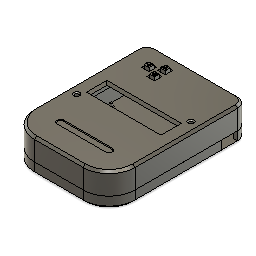
EqMountControllerCase (Autodesk Fusion 360 design; units mm, degrees)
Autodesk Fusion 360 part; units mm, degrees
sketch "Sketch1" plane through (0, 0, 0) normal (0, 1, 0) x (1, 0, 0)
  line L0 (0, 0) -> (75, 0) construction
  circle A0 centre (75, 0) radius 1.25
  line L1 (3, 0) -> (3, 29) construction
  line L2 (3, 29) -> (59, 29) construction
  line L3 (59, 29) -> (59, 65) construction
  line L4 (59, 65) -> (3, 65) construction
  line L5 (3, 65) -> (3, 29) construction
  circle A1 centre (3, 29) radius 1
  circle A2 centre (59, 29) radius 1
  circle A3 centre (59, 65) radius 1
  circle A4 centre (3, 65) radius 1
  line L6 (0, 0) -> (0, 31) construction
  line L7 (75, 0) -> (75, 31) construction
  line L8 (59, 65) -> (3, 29) construction
  line L9 (3, 65) -> (59, 29) construction
  line L10 (75, 31) -> (0, 0) construction
  line L11 (0, 31) -> (75, 0) construction
  line L12 (77.5, 33.5) -> (-2.5, 33.5) construction
  line L13 (-2.5, 33.5) -> (-2.5, -2.5) construction
  line L14 (-2.5, -2.5) -> (77.5, -2.5) construction
  line L15 (77.5, -2.5) -> (77.5, 33.5) construction
  line L16 (77.5, 33.5) -> (-2.5, -2.5) construction
  line L17 (-2.5, 33.5) -> (77.5, -2.5) construction
  line L18 (61, 67) -> (1, 67) construction
  line L19 (1, 67) -> (1, 27) construction
  line L20 (1, 27) -> (61, 27) construction
  line L21 (61, 27) -> (61, 67) construction
  line L22 (61, 67) -> (1, 27) construction
  line L23 (1, 67) -> (61, 27) construction
  line L24 (70, 8) -> (5, 8)
  line L25 (5, 8) -> (5, 23)
  line L26 (5, 23) -> (70, 23)
  line L27 (70, 23) -> (70, 8)
  line L28 (70, 8) -> (5, 23) construction
  line L29 (5, 8) -> (70, 23) construction
  line L30 (0, 70) -> (75, 70)
  line L31 (80, 65) -> (80, -30)
  line L32 (60, -50) -> (15, -50)
  line L33 (-5, -30) -> (-5, 65)
  arc A5 (80, 65) -> (75, 70) centre (75, 65) ccw
  arc A6 (0, 70) -> (-5, 65) centre (0, 65) ccw
  arc A7 (-5, -30) -> (15, -50) centre (15, -30) ccw
  arc A8 (60, -50) -> (80, -30) centre (60, -30) ccw
  arc A9 (0, 72) -> (-7, 65) centre (0, 65) ccw
  line L34 (-7, -30) -> (-7, 65)
  arc A10 (-7, -30) -> (15, -52) centre (15, -30) ccw
  line L35 (60, -52) -> (15, -52)
  arc A11 (60, -52) -> (82, -30) centre (60, -30) ccw
  line L36 (82, 65) -> (82, -30)
  arc A12 (82, 65) -> (75, 72) centre (75, 65) ccw
  line L37 (0, 72) -> (75, 72)
  arc A13 (0, 74) -> (-9, 65) centre (0, 65) ccw
  line L38 (-9, -30) -> (-9, 65)
  arc A14 (-9, -30) -> (15, -54) centre (15, -30) ccw
  line L39 (60, -54) -> (15, -54)
  arc A15 (60, -54) -> (84, -30) centre (60, -30) ccw
  line L40 (84, 65) -> (84, -30)
  arc A16 (84, 65) -> (75, 74) centre (75, 65) ccw
  line L41 (0, 74) -> (75, 74)
  line L42 (1, 67) -> (22, 67) construction
  line L43 (22, 67) -> (22, 60) construction
  line L44 (24.5, 57.5) -> (19.5, 57.5)
  line L45 (19.5, 57.5) -> (19.5, 62.5)
  line L46 (19.5, 62.5) -> (24.5, 62.5)
  line L47 (24.5, 62.5) -> (24.5, 57.5)
  line L48 (24.5, 57.5) -> (19.5, 62.5) construction
  line L49 (19.5, 57.5) -> (24.5, 62.5) construction
  line L50 (22, 67) -> (22, 50) construction
  line L51 (24.5, 47.5) -> (19.5, 47.5)
  line L52 (19.5, 47.5) -> (19.5, 52.5)
  line L53 (19.5, 52.5) -> (24.5, 52.5)
  line L54 (24.5, 52.5) -> (24.5, 47.5)
  line L55 (24.5, 47.5) -> (19.5, 52.5) construction
  line L56 (19.5, 47.5) -> (24.5, 52.5) construction
  line L57 (1, 67) -> (12, 67) construction
  line L58 (9.5, 52.5) -> (14.5, 52.5)
  line L59 (14.5, 52.5) -> (14.5, 57.5)
  line L60 (14.5, 57.5) -> (9.5, 57.5)
  line L61 (9.5, 57.5) -> (9.5, 52.5)
  line L62 (9.5, 52.5) -> (14.5, 57.5) construction
  line L63 (14.5, 52.5) -> (9.5, 57.5) construction
  circle A17 centre (3, 65) radius 2
  circle A18 centre (59, 65) radius 2
  circle A19 centre (59, 29) radius 2
  circle A20 centre (3, 29) radius 2
  circle A21 centre (75, 31) radius 3
  circle A22 centre (75, 0) radius 3
  circle A23 centre (0, 0) radius 3
  line L64 (84, 65) -> (80, 65)
  line L65 (80, 65) -> (80, 50)
  line L66 (80, 50) -> (84, 50)
  line L67 (84, 50) -> (84, 65)
  line L68 (-9, 65) -> (-5, 65)
  line L69 (-5, 65) -> (-5, 50)
  line L70 (-5, 50) -> (-9, 50)
  line L71 (-9, 50) -> (-9, 65)
  line L72 (26, 46) -> (8, 46)
  line L73 (8, 46) -> (8, 64)
  line L74 (8, 64) -> (26, 64)
  line L75 (26, 64) -> (26, 46)
  circle A24 centre (75, 31) radius 1.75
  circle A25 centre (0, 0) radius 1.75
  line L76 (8.5, 51.5) -> (15.5, 51.5)
  line L77 (15.5, 51.5) -> (15.5, 58.5)
  line L78 (15.5, 58.5) -> (8.5, 58.5)
  line L79 (8.5, 58.5) -> (8.5, 51.5)
  line L80 (25.5, 63.5) -> (25.5, 56.5)
  line L81 (25.5, 56.5) -> (18.5, 56.5)
  line L82 (18.5, 56.5) -> (18.5, 63.5)
  line L83 (18.5, 63.5) -> (25.5, 63.5)
  line L84 (25.5, 46.5) -> (18.5, 46.5)
  line L85 (18.5, 46.5) -> (18.5, 53.5)
  line L86 (18.5, 53.5) -> (25.5, 53.5)
  line L87 (25.5, 53.5) -> (25.5, 46.5)
  line L88 (9.7, 52.7) -> (14.3, 52.7)
  line L89 (14.3, 52.7) -> (14.3, 57.3)
  line L90 (14.3, 57.3) -> (9.7, 57.3)
  line L91 (9.7, 57.3) -> (9.7, 52.7)
  line L92 (24.3, 57.7) -> (19.7, 57.7)
  line L93 (19.7, 57.7) -> (19.7, 62.3)
  line L94 (19.7, 62.3) -> (24.3, 62.3)
  line L95 (24.3, 62.3) -> (24.3, 57.7)
  line L96 (24.3, 47.7) -> (19.7, 47.7)
  line L97 (19.7, 47.7) -> (19.7, 52.3)
  line L98 (19.7, 52.3) -> (24.3, 52.3)
  line L99 (24.3, 52.3) -> (24.3, 47.7)
  line L100 (9.7, 55) -> (13.15, 53.0081)
  line L101 (13.15, 53.0081) -> (13.15, 56.9919)
  line L102 (13.15, 56.9919) -> (9.7, 55)
  line L103 (22, 62.3) -> (20.0081, 58.85)
  line L104 (20.0081, 58.85) -> (23.9919, 58.85)
  line L105 (23.9919, 58.85) -> (22, 62.3)
  line L106 (22, 47.7) -> (23.9919, 51.15)
  line L107 (23.9919, 51.15) -> (20.0081, 51.15)
  line L108 (20.0081, 51.15) -> (22, 47.7)
  line L109 (76.25, 32.25) -> (73.75, 32.25)
  line L110 (73.75, 32.25) -> (73.75, 29.75)
  line L111 (73.75, 29.75) -> (76.25, 29.75)
  line L112 (76.25, 29.75) -> (76.25, 32.25)
  line L113 (76.25, 32.25) -> (73.75, 29.75) construction
  line L114 (73.75, 32.25) -> (76.25, 29.75) construction
  line L115 (1.25, 1.25) -> (-1.25, 1.25)
  line L116 (-1.25, 1.25) -> (-1.25, -1.25)
  line L117 (-1.25, -1.25) -> (1.25, -1.25)
  line L118 (1.25, -1.25) -> (1.25, 1.25)
  line L119 (1.25, 1.25) -> (-1.25, -1.25) construction
  line L120 (-1.25, 1.25) -> (1.25, -1.25) construction
  dimension "d2" = 75
  dimension "d3" = 2.5
  dimension "d4" = 29
  dimension "d5" = 56
  dimension "d6" = 36
  dimension "d7" = 2
  dimension "d8" = 2
  dimension "d9" = 2
  dimension "d10" = 2
  dimension "d16" = 31
  dimension "d17" = 80
  dimension "d18" = 36
  dimension "d19" = 60
  dimension "d20" = 40
  dimension "d21" = 65
  dimension "d22" = 15
  dimension "d23" = 85
  dimension "d24" = 120
  dimension "d25" = 5
  dimension "d26" = 5
  dimension "d27" = 20
  dimension "d28" = 20
  dimension "d29" = 2
  dimension "d30" = 4
  dimension "d31" = 21
  dimension "d32" = 7
  dimension "d33" = 5
  dimension "d34" = 5
  dimension "d35" = 17
  dimension "d36" = 5
  dimension "d37" = 5
  dimension "d38" = 11
  dimension "d39" = 12
  dimension "d40" = 5
  dimension "d41" = 5
  dimension "d43" = 4
  dimension "d44" = 15
  dimension "d80" = 3.5
  dimension "d81" = 3.5
  dimension "d92" = 1
  dimension "d93" = -1
  dimension "d94" = -1
  dimension "d95" = -0.2
  dimension "d96" = 0.2
  dimension "d97" = 0.2
  dimension "d112" = 2.5
  dimension "d113" = 2.5
  dimension "d114" = 2.5
  dimension "d115" = 2.5
  measures "d3" diameter of A0
  measures "d5" distance of L0.start
  measures "d7" diameter of A1
  measures "d8" diameter of A2
  measures "d9" diameter of A3
  measures "d10" diameter of A4
  measures "d21" distance of L0.start
  measures "d23" distance of L0.start
  measures "d25" radius of A5
  measures "d26" radius of A6
  measures "d27" radius of A7
  measures "d28" radius of A8
  measures "d33" distance of L0.start
  measures "d37" distance of L0.start
  measures "d38" distance of L0.start
  measures "d80" diameter of A24
  measures "d81" diameter of A25
  measures "d92" distance of L58
  measures "d94" distance of L51
  measures "d95" distance of L58
  measures "d96" distance of L44
  measures "d97" distance of L51
extrude "Extrude1" add sketch "Sketch1" along normal blind 15 contours L30 A5 A6 A9 A12 L37 L64 L68 | L31 L32 L33 A7 A8 L34 A10 L35 A11 L36 L66 L70 makes body 1 at (80, 5, -23.3333) makes body 2 at (25, 5, -72)
extrude "Extrude2" add sketch "Sketch1" along normal blind 2 contours L33 L34 L68 L69 L70 | L31 L36 L64 L65 L66 | L34 L38 L68 L70 L71 | L36 L40 L64 L66 L67 bodies 1 2
extrude "Extrude3" add sketch "Sketch1" along normal blind 10 contours A9 A12 L37 A13 A16 L41 L64 L68 | L34 A10 L35 A11 L36 L38 A14 L39 A15 L40 L66 L70 bodies 1
extrude "Extrude4" add sketch "Sketch1" along normal blind 18 separate body contours A21 | A23 | A24 L112 | A24 L109 L110 L111 L112 | A24 L109 L112 | A24 L111 L112 | A24 L109 | A24 L111 | A24 L109 L110 | A24 L110 L111 | A24 L110 | A25 L118 | A25 L115 L116 L117 L118 | A25 L115 L118 | A25 L117 L118 | A25 L115 | A25 L117 | A25 L115 L116 | A25 L116 L117 | A25 L116 makes body 3 at (2.9963, 12, 0.1495) makes body 4 at (74.9252, 12, -33.9991)
extrude "Extrude5" add sketch "Sketch1" along normal blind 18 separate body contours A22 makes body 5
extrude "Extrude18" cut sketch "Sketch1" along normal blind 24 and the other way blind -5 contours A24 L109 L110 L111 L112 | A25 L115 L116 L117 L118 bodies 4 3
extrude "Extrude13" add sketch "Sketch1" along normal blind 21 contours A0 bodies 5
extrude "Extrude6" add sketch "Sketch1" along normal blind 10 separate body contours A1 | A2 | A3 | A4 makes body 6 at (2.0309, 6.6667, -65.2468) makes body 7 at (59.9691, 6.6667, -65.2468) makes body 8 at (3.9988, 6.6667, -28.9502) makes body 9 at (59.6617, 6.6667, -29.7498)
extrude "Extrude7" add sketch "Sketch1" along normal blind 7 contours A17 | A18 | A19 | A20 bodies 6 7 8 9
extrude "Extrude8" add sketch "Sketch1" along normal blind 2 contours L24 L25 L26 L27 | L30 L31 L32 L33 A5 A6 A7 A8 L65 L69 | L44 L45 L46 L47 | L51 L52 L53 L54 | L58 L59 L60 L61 | L72 L73 L74 L75 | L76 L77 L78 L79 | L80 L81 L82 L83 | L84 L85 L86 L87 | L100 L101 L102 | L88 L89 L90 L91 | L103 L104 L105 | L92 L93 L94 L95 | L106 L107 L108 | L96 L97 L98 L99 bodies 1 4 3 5 6 7 8 9
extrude "Extrude9" add sketch "Sketch1" along normal blind 30 and the other way blind -10 separate body contours A9 A12 L37 A13 A16 L41 L64 L68 | L34 L38 L68 L70 L71 | L36 L40 L64 L66 L67 | L34 A10 L35 A11 L36 L38 A14 L39 A15 L40 L66 L70 makes body 10
extrude "Extrude10" add sketch "Sketch1" along normal blind 30 and the other way blind -15 contours L30 A5 A6 A9 A12 L37 L64 L68 | L33 L34 L68 L69 L70 | L31 L36 L64 L65 L66 | L31 L32 L33 A7 A8 L34 A10 L35 A11 L36 L66 L70 bodies 10
extrude "Extrude11" add sketch "Sketch1" along normal blind 30 and the other way blind -28 contours A0 | A1 | A2 | A3 | A4 | L30 L31 L32 L33 A5 A6 A7 A8 L65 L69 | A17 | A18 | A19 | A20 | A21 | A22 | A23 | L72 L73 L74 L75 | A24 L109 L112 | A24 L111 L112 | A24 L109 L110 | A24 L110 L111 | A25 L115 L118 | A25 L117 L118 | A25 L115 L116 | A25 L116 L117 | L76 L77 L78 L79 | L80 L81 L82 L83 | L84 L85 L86 L87 bodies 10
chamfer "Chamfer1" distance 2 angle 45 4 edges at (5, 30, -15.5) (37.5, 30, -23) (37.5, 30, -8) (70, 30, -15.5) on bodies 10
chamfer "Chamfer2" distance 2 angle 45 8 edges at (81.364, 30, -71.364) (37.5, 30, -74) (-6.364, 30, -71.364) (-9, 30, -17.5) (-1.9706, 30, 46.9706) (37.5, 30, 54) (76.9706, 30, 46.9706) (84, 30, -17.5) on bodies 10
chamfer "Chamfer3" distance 2 angle 45 8 edges at (-6.364, 0, -71.364) (37.5, 0, -74) (81.364, 0, -71.364) (84, 0, -17.5) (76.9706, 0, 46.9706) (37.5, 0, 54) (-1.9706, 0, 46.9706) (-9, 0, -17.5) on bodies 1
extrude "Extrude12" add sketch "Sketch1" along normal blind 28 and the other way blind -23 contours L72 L73 L74 L75 | L76 L77 L78 L79 | L80 L81 L82 L83 | L84 L85 L86 L87 bodies 10
extrude "Extrude14" add sketch "Sketch1" along normal blind 28 and the other way blind -20 contours A21 | A23 | A24 L109 L112 | A24 L111 L112 | A24 L109 L110 | A24 L110 L111 | A25 L115 L118 | A25 L117 L118 | A25 L115 L116 | A25 L116 L117 bodies 10
chamfer "Chamfer4" distance 1 angle 45 14 edges at (-1.6316, 30, -0.6328) (73.3684, 30, -31.6328) (24.5, 30, -60) (22, 30, -62.5) (19.5, 30, -60) (22, 30, -57.5) (12, 30, -57.5) (9.5, 30, -55) (12, 30, -52.5) (14.5, 30, -55) (19.5, 30, -50) (22, 30, -52.5) (22, 30, -47.5) (24.5, 30, -50) on bodies 10
chamfer "Chamfer5" distance 2 angle 45 7 edges at (1.1353, 2, -29.7232) (1.1353, 2, -65.7232) (57.1353, 2, -65.7232) (57.1353, 2, -29.7232) (72.203, 2, -1.0848) (-2.797, 2, -1.0848) (72.203, 2, -32.0848) on bodies 1
chamfer "Chamfer6" distance 1 angle 45 8 edges at (-7, 15, -10) (-0.5563, 15, 45.5563) (37.5, 15, 52) (75.5563, 15, 45.5563) (82, 15, -10) (79.9497, 15, -69.9497) (37.5, 15, -72) (-4.9497, 15, -69.9497) on bodies 1 2
chamfer "Chamfer7" distance 1 angle 45 8 edges at (37.5, 10, -72) (79.9497, 10, -69.9497) (82, 10, -17.5) (75.5563, 10, 45.5563) (37.5, 10, 52) (-0.5563, 10, 45.5563) (-7, 10, -17.5) (-4.9497, 10, -69.9497) on bodies 10
extrude "Extrude15" add sketch "Sketch1" along normal blind 32 and the other way blind -19 separate body contours L100 L101 L102 | L88 L89 L90 L91 | L103 L104 L105 | L92 L93 L94 L95 | L106 L107 L108 | L96 L97 L98 L99 makes body 11 at (9.7, 23.3333, -55.7667) makes body 12 at (19.7, 23.3333, -49.2333) makes body 13 at (19.7, 23.3333, -59.2333)
extrude "Extrude16" add sketch "Sketch1" along normal blind 19 and the other way blind -14 contours L44 L45 L46 L47 | L51 L52 L53 L54 | L58 L59 L60 L61 | L76 L77 L78 L79 | L80 L81 L82 L83 | L84 L85 L86 L87 | L100 L101 L102 | L88 L89 L90 L91 | L103 L104 L105 | L92 L93 L94 L95 | L106 L107 L108 | L96 L97 L98 L99 bodies 11 12 13
chamfer "Chamfer8" distance 1 angle 45 36 edges at (15.5, 19, -55) (12, 19, -58.5) (15.5, 16.5, -58.5) (12, 14, -58.5) (8.5, 16.5, -58.5) (8.5, 19, -55) (8.5, 14, -55) (8.5, 16.5, -51.5) (12, 19, -51.5) (15.5, 16.5, -51.5) (12, 14, -51.5) (15.5, 14, -55) (25.5, 19, -50) (22, 19, -46.5) (22, 14, -46.5) (25.5, 14, -50) (22, 19, -53.5) (22, 14, -53.5) (18.5, 19, -50) (18.5, 14, -50) (18.5, 16.5, -53.5) (18.5, 16.5, -46.5) (25.5, 16.5, -46.5) (25.5, 16.5, -53.5) (22, 19, -56.5) (25.5, 19, -60) (22, 19, -63.5) (25.5, 14, -60) (22, 14, -63.5) (18.5, 19, -60) (18.5, 14, -60) (18.5, 16.5, -63.5) (25.5, 16.5, -63.5) (18.5, 16.5, -56.5) (25.5, 16.5, -56.5) (22, 14, -56.5) on bodies 11 12 13
extrude "Extrude17" add sketch "Sketch1" along normal blind 32 and the other way blind -33 contours L100 L101 L102 | L103 L104 L105 | L106 L107 L108 bodies 11 12 13
chamfer "Chamfer9" distance 0.4 angle 45 9 edges at (11.425, 33, -55.9959) (11.425, 33, -54.0041) (13.15, 33, -55) (21.0041, 33, -49.425) (22, 33, -51.15) (22.9959, 33, -49.425) (22, 33, -58.85) (21.0041, 33, -60.575) (22.9959, 33, -60.575) on bodies 11 12 13
sketch "Sketch2" plane through (0, 0, 0) normal (0, 1, 0) x (1, 0, 0)
  line L0 (17.5, -30) -> (17.5, 50)
  arc A0 (17.5, 50) -> (12.5, 50) centre (15, 50) ccw
  line L1 (12.5, 50) -> (12.5, -30)
  arc A1 (12.5, -30) -> (17.5, -30) centre (15, -30) ccw
  line L2 (15, -30) -> (15, 50) construction
  line L3 (26, 46) -> (8, 46)
  line L4 (62.5, -30) -> (62.5, 50)
  arc A2 (62.5, 50) -> (57.5, 50) centre (60, 50) ccw
  line L5 (57.5, 50) -> (57.5, -30)
  arc A3 (57.5, -30) -> (62.5, -30) centre (60, -30) ccw
  line L6 (60, -30) -> (60, 50) construction
  line L7 (61, 27) -> (61, 67)
  line L8 (15, -32.5) -> (60, -32.5)
  arc A4 (60, -32.5) -> (60, -27.5) centre (60, -30) ccw
  line L9 (60, -27.5) -> (15, -27.5)
  arc A5 (15, -27.5) -> (15, -32.5) centre (15, -30) ccw
  line L10 (15, -30) -> (60, -30) construction
  dimension "d120" = 5
  dimension "d121" = 5
  measures "d120" diameter of A0
  measures "d121" diameter of A2
extrude "Extrude19" cut sketch "Sketch2" along normal blind 0.6 contours L0 A1 L9 A5 | L0 L1 L3 L9 A5 | L0 A0 L1 L3 | L5 A3 A4 L9 | L4 A2 L5 A4 L9 bodies 1
chamfer "Chamfer10" distance 0.6 angle 45 8 edges at (57.5, 0, -10) (60, 0, 32.5) (62.5, 0, -10) (60, 0, -52.5) (12.5, 0, -10) (15, 0, 32.5) (17.5, 0, -10) (15, 0, -52.5) on bodies 1
extrude "Extrude20" cut sketch "Sketch2" along normal blind 37 and the other way blind -29.4 contours L0 A1 L9 A5 | L0 A1 L5 A3 L8 L9 | L5 A3 A4 L9 bodies 10
chamfer "Chamfer11" distance 0.6 angle 45 4 edges at (37.5, 30, 32.5) (12.5, 30, 30) (37.5, 30, 27.5) (62.5, 30, 30) on bodies 10
named bodies: "BoxBottom", "BoxTop", "ButtonNext", "ButtonDown", "ButtonUp"
